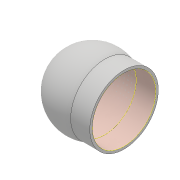
# Autodesk Inventor part: GradFormerBase_190719_v03_fromdims
Saved by Autodesk Inventor 2018 (Build 220112000, 112)
## iProperties
Created: 2019-07-19
Part Number: GradFormerBase_190719_v03_fromdims
Material: Generic
Document SubType Name: Modeling
Designer: pm589
Density: 1 g/cm^3
Appearance: Default
Author: pm589
Autodesk Inventor part; units mm, degrees
ref_plane "YZ Plane" through (0, 0, 0) normal (1, 0, 0) x (0, 1, 0)
ref_plane "XZ Plane" through (0, 0, 0) normal (0, 1, 0) x (-1, 0, 0)
ref_plane "XY Plane" through (0, 0, 0) normal (0, 0, 1) x (1, 0, 0)
sketch "Sketch1" plane through (0, 0, 0) normal (0, 0, 1) x (1, 0, 0)
  line L0 (177.8, 183.889) -> (68.6887, 183.889)
  arc A0 (68.6887, 183.889) -> (-196.299, 0) centre (0, 0) ccw
  line L1 (-196.299, 0) -> (0, 0) construction
  line L2 (0, 0) -> (68.6887, 183.889) construction
  line L3 (-328.8502, 0) -> (262.2417, 0) projected
  line L4 (0, 303.8589) -> (0, -50.6431) projected
  dimension "d0" = 177.8
  dimension "d1" = 183.889
  dimension "d2" = 196.299
  constraints: 6 end point, 2 point on circle, 1 centre point, 1 coincident, 1 collinear, 1 horizontal
  measures "d0" distance from line of L4 L0.start
  measures "d1" distance between parallel lines of L3 L0
  measures "d2" radius of A0
surface revolve "RevolutionSrf1" sketch "Sketch1" angle 360 about axis through (0, 0, 0) along (1, 0, 0) shown no curves L0 A0
thicken "Thicken1" operation new thickness 9 both sides no extend neighbours no toward (0.0039661, 0.5837391, -0.8119316) faces at (0.7785, 114.5874, -159.3814) (141.4296, -107.8317, -148.9547)
thicken "Thicken2" operation add thickness 5 both sides no extend neighbours no toward (0, 0.5863955, 0.8100249) faces at (141.4296, -107.8317, -148.9547) (0.7785, 114.5874, -159.3814)
surface_offset "OffsetSrf1"
equation "\"d0\" = gfbase_xmax"
equation "\"d1\" = 0.5 * gfbase_dmid_cyl"
equation "\"d2\" = 0.5 * gfbase_dmid_sph"
equation "\"d4\" = gfbase_t_outer"
equation "\"d5\" = gfbase_t_outer"
equation "\"d6\" = gfbase_t_inner"
equation "\"d7\" = gfbase_t_inner"
equation "\"d8\" = gfbase_b0magtol"
equation "\"d9\" = gfbase_b0magtol"
equation "\"gfbase_t_inner\" = 5"
equation "\"gfbase_t_outer\" = 9"
equation "\"gfbase_xmax\" = 177.8"
equation "\"gfbase_dmid_sph\" = 392.598"
equation "\"gfbase_dmid_cyl\" = 367.778"
equation "\"gfbase_b0magtol\" = 0.5"
equation "\"gfbase_pegtol\" = 0.5"
equation "\"gfbase_magrail_offset\" = 1"
body "Solid1"
body "Srf1"
body "Srf2"
